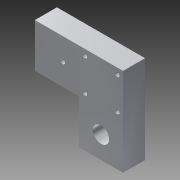
# Autodesk Inventor part: wooden1
Saved by Autodesk Inventor 2015 (Build 190159000, 159)
## iProperties
Created: 2016-04-26
Part Number: wooden1
Material: Aluminum 6061
Document SubType Name: Modeling
Designer: Kostya
Density: 2.7 g/cm^3
Appearance: Aluminum - Flat
Author: Kostya
Autodesk Inventor part; units mm, degrees
ref_plane "YZ Plane" through (0, 0, 0) normal (1, 0, 0) x (0, 1, 0)
ref_plane "XZ Plane" through (0, 0, 0) normal (0, 1, 0) x (-1, 0, 0)
ref_plane "XY Plane" through (0, 0, 0) normal (0, 0, 1) x (1, 0, 0)
sketch "Sketch1" plane through (0, 0, 0) normal (0, 1, 0) x (-1, 0, 0)
  line L0 (0, 0) -> (60, 0)
  line L1 (60, 0) -> (60, -30)
  line L2 (60, -30) -> (30, -30)
  line L3 (30, -30) -> (30, -60)
  line L4 (30, -60) -> (0, -60)
  line L5 (0, -60) -> (0, 0)
  dimension "d0" = 60
  dimension "d1" = 30
  dimension "d2" = 30
  dimension "d3" = 30
  dimension "d4" = 30
  constraints: 12 end point, 4 perpendicular, 1 horizontal
  measures "d0" distance of L0.start L0.end
  measures "d1" distance of L0.end L1.end
  measures "d2" distance of L1.end L2.end
  measures "d3" distance of L2.end L3.end
  measures "d4" distance of L3.end L4.end
extrude "Extrusion1" add sketch "Sketch1" along normal blind 15
sketch "Sketch13" plane through (0, 0, 0) normal (0, -1, 0) x (1, 0, 0)
  circle A0 centre (-4, -4) radius 1.5
  circle A1 centre (-26, -4) radius 1.5
  circle A2 centre (-4, -26) radius 1.5
  circle A3 centre (-26, -26) radius 1.5
  point P0 (0, 0)
  dimension "d55" = 3
  dimension "d56" = 3
  dimension "d57" = 3
  dimension "d58" = 3
  constraints: 4 centre point
  measures "d55" diameter of A0
  measures "d56" diameter of A1
  measures "d57" diameter of A2
  measures "d58" diameter of A3
extrude "Extrusion7" cut sketch "Sketch13" against normal up to next
sketch "Sketch14" plane through (0, 0, 0) normal (0, -1, 0) x (1, 0, 0)
  circle A0 centre (-41, -15) radius 1.5
  line L0 (-60, 0) -> (-60, -30) projected
  line L1 (0, 0) -> (-60, 0) projected
  circle A1 centre (-15, -45) radius 3
  line L2 (-30, -60) -> (0, -60) projected
  line L3 (-30, -30) -> (-30, -60) projected
  dimension "d61" = 3
  dimension "d62" = 19
  dimension "d63" = 15
  dimension "d64" = 6
  dimension "d65" = 15
  dimension "d66" = 15
  constraints: 2 centre point
  measures "d61" diameter of A0
  measures "d62" distance from line of L0 A0.centre
  measures "d63" distance from line of L1 A0.centre
  measures "d64" diameter of A1
  measures "d65" distance from line of L2 A1.centre
  measures "d66" distance from line of L3 A1.centre
extrude "Extrusion8" cut sketch "Sketch14" against normal up to next
sketch "Sketch15" plane through (0, 0, 0) normal (0, -1, 0) x (1, 0, 0)
  circle A0 centre (-15, -45) radius 5.5
  point P0 (0, 0)
  dimension "d69" = 11
  constraints: 1 centre point
  measures "d69" diameter of A0
extrude "Extrusion9" cut sketch "Sketch15" against normal blind 11
sketch "Sketch2" plane through (0, 0, 0) normal (0, -1, 0) x (1, 0, 0)
  point P0 (-15, -45)
sketch "Sketch3" plane through (0, 15, 0) normal (0, 1, 0) x (1, 0, 0)
  point P0 (-45, 15)
body "Solid1"
